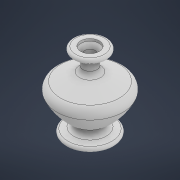
# Autodesk Inventor part: Pieza de practica 13
Saved by Autodesk Inventor 2022 (Build 260153000, 153)
## iProperties
Created: 2022-08-24
Part Number: Pieza de practica 13
Material: Genérico
Document SubType Name: Modeling
Designer: aleon
Density: 1 g/cm^3
Appearance: Valor por defecto
Author: aleon
Autodesk Inventor part; units mm, degrees
ref_plane "YZ Plane" through (0, 0, 0) normal (1, 0, 0) x (0, 1, 0)
ref_plane "XZ Plane" through (0, 0, 0) normal (0, 1, 0) x (-1, 0, 0)
ref_plane "XY Plane" through (0, 0, 0) normal (0, 0, 1) x (1, 0, 0)
sketch "Boceto2" plane through (0, 0, 0) normal (1, 0, 0) x (0, 1, 0)
  line L0 (0, 0) -> (160, 0)
  arc A0 (138.2668, 15) -> (150.0785, 29.1176) centre (138.2668, 27) ccw
  line L1 (138.2668, 15) -> (124.5668, 15)
  arc A1 (113.5974, 22.1347) -> (124.5668, 15) centre (124.5668, 27) ccw
  line L2 (113.5974, 22.1347) -> (96.0259, 61.7513)
  arc A2 (96.0259, 61.7513) -> (74.2791, 69.5922) centre (81.4, 55.2642) ccw
  arc A3 (74.2791, 69.5922) -> (28.9728, 31.3484) centre (129.8222, -42.1665) ccw
  arc A4 (12.9956, 34.3623) -> (28.9728, 31.3484) centre (21.7, 36.65) ccw
  line L3 (0, 0) -> (0, 45.1139)
  line L4 (74.2791, 69.5922) -> (34.1, 0)
  line L5 (12.9956, 34.3623) -> (9.8358, 46.3849)
  arc A5 (9.8358, 46.3849) -> (0, 45.1139) centre (5, 45.1139) ccw
  arc A6 (160, 30) -> (150.0785, 29.1176) centre (155, 30) ccw
  line L6 (4.4, 45.1139) -> (4.4, 0)
  arc A7 (147.0526, 10.6) -> (155.2933, 19.5) centre (138.2668, 27) ccw
  line L7 (147.0526, 10.6) -> (124.5668, 10.6)
  arc A8 (109.5752, 20.3507) -> (124.5668, 10.6) centre (124.5668, 27) ccw
  line L8 (109.5752, 20.3507) -> (92.0038, 59.9674)
  arc A9 (92.0038, 59.9674) -> (76.2373, 65.652) centre (81.4, 55.2642) ccw
  arc A10 (76.2373, 65.652) -> (32.5284, 28.7566) centre (129.8222, -42.1665) ccw
  arc A11 (8.7401, 33.2438) -> (32.5284, 28.7566) centre (21.7, 36.65) ccw
  line L9 (8.7401, 33.2438) -> (5.5803, 45.2664)
  arc A12 (5.5803, 45.2664) -> (4.4, 45.1139) centre (5, 45.1139) ccw
  line L10 (160, 30) -> (160, 19.5)
  line L11 (160, 19.5) -> (155.2933, 19.5)
  dimension "d6" = 12
  dimension "d7" = 13.7
  dimension "d8" = 16
  dimension "d9" = 124.8
  dimension "d10" = 9
  dimension "d12" = 34.1
  dimension "d13" = 60
  dimension "d14" = 59.7
  dimension "d15" = 21.7
  dimension "d16" = 5
  dimension "d17" = 36.65
  dimension "d18" = 12
  dimension "d19" = 5
  dimension "d22" = 4.4
  dimension "d23" = 8.9
  dimension "d24" = 10.5
  dimension "d25" = 30
  dimension "d26" = 160
  constraints: 26 point on circle, 24 end point, 13 centre point, 11 tangent, 3 horizontal, 2 point on line, 2 vertical, 1 perpendicular, 1 vertical alignment, 7 other
  measures "d6" radius of A1
  measures "d7" distance of L1.start L1.end
  measures "d8" radius of A2
  measures "d9" radius of A3
  measures "d10" radius of A4
  measures "d12" distance of L0.start L4.end
  measures "d13" angle of L4 L0
  measures "d14" horizontal distance of A4.centre A2.centre
  measures "d15" horizontal distance of L0.start A4.centre
  measures "d16" radius of A5
  measures "d17" vertical distance of A4.centre L0.start
  measures "d18" radius of A0
  measures "d19" radius of A6
  measures "d22" distance between parallel lines of L3 L6
  measures "d23" vertical distance of L10.end L7.start
  measures "d24" distance from line of A6.centre L11
  measures "d25" distance from line of A6.centre L0
  measures "d26" distance of L0.start L0.end
revolve "Revolución3" add sketch "Boceto2" angle 360 about axis through (0, 0, 0) along (0, 1, 0) contours L3 A5 L5 A4 A3 L4 A10 A11 L9 A12 L6 L0 | L4 A2 L2 A1 L1 A0 A6 L10 L11 A7 L7 A8 L8 A9 A10
